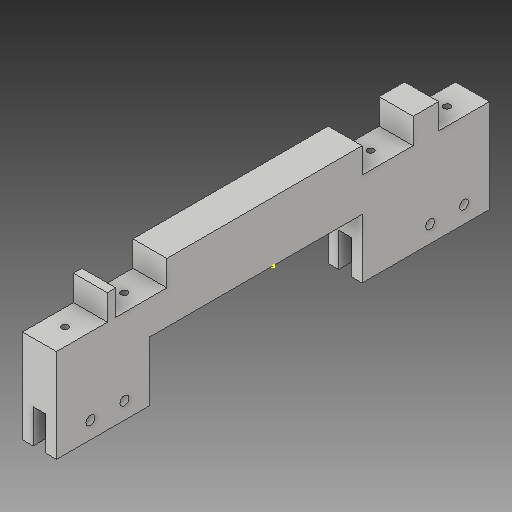
# Autodesk Inventor part: RailSlideLeftSide
Saved by Autodesk Inventor 2017 SP1 (Build 210196100, 196)
## iProperties
Created: 2016-02-14
Part Number: RailSlideLeftSide
Material: Generic
Document SubType Name: Modeling
Designer: steele
Density: 1 g/cm^3
Appearance: Default
Author: steele
Autodesk Inventor part; units mm, degrees
ref_plane "YZ Plane" through (0, 0, 0) normal (1, 0, 0) x (0, 1, 0)
ref_plane "XZ Plane" through (0, 0, 0) normal (0, 1, 0) x (-1, 0, 0)
ref_plane "XY Plane" through (0, 0, 0) normal (0, 0, 1) x (1, 0, 0)
sketch "Sketch1" plane through (0, 0, 0) normal (1, 0, 0) x (0, 1, 0)
  line L0 (-44.45, 161.925) -> (-44.45, -161.925)
  line L1 (-44.45, -161.925) -> (44.45, -161.925)
  line L2 (44.45, -161.925) -> (44.45, 161.925)
  line L3 (44.45, 161.925) -> (-44.45, 161.925)
  line L4 (-44.45, 161.925) -> (44.45, -161.925) construction
  line L5 (-44.45, -161.925) -> (44.45, 161.925) construction
  point P0 (0, 0)
  dimension "d0" = 323.85
  dimension "d1" = 88.9
  constraints: 12 end point, 2 midpoint, 2 parallel, 1 perpendicular, 1 vertical
  measures "d0" distance of L1.end L2.end
  measures "d1" distance of L2.end L0.start
extrude "Extrusion1" add sketch "Sketch1" along normal mid plane 25.4
sketch "Sketch2" plane through (12.7, 0, 0) normal (1, 0, 0) x (0, 0, -1)
  line L0 (-161.925, -44.45) -> (161.925, -44.45) projected
  line L1 (-92.075, -44.45) -> (66.675, -44.45)
  line L2 (66.675, -44.45) -> (66.675, 0)
  line L3 (66.675, 0) -> (-92.075, 0)
  line L4 (-92.075, 0) -> (-92.075, -44.45)
  line L5 (-161.925, 44.45) -> (-161.925, -44.45) projected
  point P0 (0, 0)
  dimension "d4" = 158.75
  dimension "d5" = 44.45
  dimension "d6" = 69.85
  constraints: 8 end point, 2 parallel, 1 horizontal, 1 perpendicular, 1 point on line
  measures "d4" distance of L2.end L3.end
  measures "d5" distance between parallel lines of L0 L3
  measures "d6" distance between parallel lines of L4 L5
extrude "Extrusion2" cut sketch "Sketch2" against normal through all
sketch "Sketch4" plane through (-12.7, -44.45, 161.925) normal (0, 0, 1) x (1, 0, 0)
  line L0 (7.9375, 0) -> (17.4625, 0)
  line L1 (17.4625, 0) -> (17.4625, 25.4)
  line L2 (17.4625, 25.4) -> (7.9375, 25.4)
  line L3 (7.9375, 25.4) -> (7.9375, 0)
  line L4 (25.4, 0) -> (0, 0) projected
  point P0 (12.7, 44.45)
  dimension "d11" = 4.7625
  dimension "d12" = 4.7625
  dimension "d13" = 25.4
  constraints: 8 end point, 2 parallel, 1 collinear, 1 horizontal, 1 perpendicular
  measures "d11" distance from line of point (12.7, 44.45) L3
  measures "d12" distance from line of point (12.7, 44.45) L1
  measures "d13" distance of L2.end L0.start
extrude "Extrusion3" cut sketch "Sketch4" against normal through all
sketch "Sketch6" plane through (12.7, 0, 0) normal (1, 0, 0) x (0, 0, -1)
  point P0 (0, 0)
sketch "Sketch7" plane through (12.7, 0, 0) normal (1, 0, 0) x (0, 0, -1)
  line L0 (-161.925, 44.45) -> (-161.925, -44.45) projected
  line L1 (-161.925, -44.45) -> (-161.925, 44.45) construction
  line L2 (-161.925, -31.75) -> (161.925, -31.75) construction
  line L3 (161.925, 44.45) -> (161.925, -44.45) construction
  point P0 (0, 0)
  point P1 (-136.525, -31.75)
  point P2 (-111.125, -31.75)
  point P3 (117.475, -31.75)
  point P4 (142.875, -31.75)
  dimension "d16" = 12.7
  dimension "d17" = 25.4
  dimension "d18" = 25.4
  dimension "d19" = 279.4
  dimension "d20" = 25.4
  constraints: 6 point on line, 2 end point, 1 horizontal
  measures "d16" distance from line of L2 L0.end
  measures "d17" distance of point (-111.125, -31.75) point (-136.525, -31.75)
  measures "d18" distance from line of L0 point (-136.525, -31.75)
  measures "d19" distance from line of point (117.475, -31.75) L0
  measures "d20" distance of point (142.875, -31.75) point (117.475, -31.75)
hole "Hole1" at (12.7, -31.75, 136.525) at (12.7, -31.75, 111.125) at (12.7, -31.75, -117.475) at (12.7, -31.75, -142.875) direction (-1, 0, 0) diameter 6.7564 end through all clearance for "Flat Head Machine Screw (82)" size "1/4" standard "Ansi Unified Screw Threads"
sketch "Sketch8" plane through (12.7, 0, 0) normal (1, 0, 0) x (0, 0, -1)
  line L0 (-161.925, 44.45) -> (-161.925, -44.45) projected
  line L1 (-161.925, 25.4) -> (-123.825, 25.4)
  line L2 (-123.825, 25.4) -> (-123.825, 44.45)
  line L3 (-123.825, 44.45) -> (-161.925, 44.45)
  line L4 (-161.925, 44.45) -> (-161.925, 25.4)
  line L5 (161.925, 44.45) -> (-161.925, 44.45) projected
  line L6 (161.925, 44.45) -> (161.925, -44.45) projected
  line L7 (161.925, 25.4) -> (123.825, 25.4)
  line L8 (123.825, 25.4) -> (123.825, 44.45)
  line L9 (123.825, 44.45) -> (161.925, 44.45)
  line L10 (161.925, 44.45) -> (161.925, 25.4)
  line L11 (-117.475, 44.45) -> (-79.375, 44.45)
  line L12 (-79.375, 44.45) -> (-79.375, 25.4)
  line L13 (-79.375, 25.4) -> (-117.475, 25.4)
  line L14 (-117.475, 25.4) -> (-117.475, 44.45)
  line L15 (104.775, 25.4) -> (66.675, 25.4)
  line L16 (66.675, 25.4) -> (66.675, 44.45)
  line L17 (66.675, 44.45) -> (104.775, 44.45)
  line L18 (104.775, 44.45) -> (104.775, 25.4)
  point P0 (0, 0)
  dimension "d28" = 38.1
  dimension "d29" = 19.05
  dimension "d30" = 6.35
  dimension "d31" = 146.05
  constraints: 32 end point, 8 parallel, 7 collinear, 5 point on line, 4 horizontal, 4 perpendicular
  measures "d28" distance of L1.start L1.end
  measures "d29" distance of L1.end L2.end
  measures "d30" distance between parallel lines of L14 L2
  measures "d31" distance between parallel lines of L16 L12
extrude "Extrusion4" cut sketch "Sketch8" against normal through all
sketch "Sketch9" plane through (12.7, 25.4, 161.925) normal (0, 1, 0) x (1, 0, 0)
  line L0 (-17.4625, 0) -> (-7.9375, 0) construction
  line L1 (-12.7, 0) -> (-12.7, 323.226) construction
  line L2 (0, 0) -> (-25.4, 0) construction
  line L3 (0, 44.45) -> (-25.4, 44.45) construction
  line L4 (0, 228.6) -> (-25.4, 228.6) construction
  line L5 (0, 285.75) -> (-25.4, 285.75) construction
  point P0 (-12.7, 161.925)
  point P1 (-12.7, 19.05)
  point P2 (-12.7, 63.5)
  point P3 (-12.7, 247.65)
  point P4 (-12.7, 304.8)
  dimension "d34" = 19.05
  dimension "d35" = 19.05
  dimension "d36" = 19.05
  dimension "d37" = 19.05
  constraints: 4 point on line, 2 end point, 1 midpoint, 1 vertical
  measures "d34" distance from line of point (-12.7, 19.05) L2
  measures "d35" distance from line of point (-12.7, 63.5) L3
  measures "d36" distance from line of point (-12.7, 247.65) L4
  measures "d37" distance from line of point (-12.7, 304.8) L5
hole "Hole2" at (0, 25.4, 142.875) at (0, 25.4, 98.425) at (0, 25.4, -85.725) at (0, 25.4, -142.875) direction (0, -1, 0) diameter 4.9784 depth 31.75 tip angle 118 thread size "1/4-20 UNC" class "2B" standard "ANSI Unified Screw Threads"
equation "\"d0\" = RailSlideTotalLength"
equation "\"d1\" = RailSlideTotalHeight"
equation "\"d2\" = RailSlideTotalWidth"
equation "\"d4\" = WidthOfCutoutForTransmission"
equation "\"d5\" = heigthOfCutoutForTransmission"
equation "\"d6\" = distanceFromRearToStartOfTransmissionCutout"
equation "\"d7\" = RailSlideTotalWidth"
equation "\"d11\" = 0.5 * cutoutWidth"
equation "\"d12\" = 0.5 * cutoutWidth"
equation "\"d13\" = cutoutHeight"
equation "\"d14\" = RailSlideTotalWidth"
equation "\"d32\" = RailSlideTotalWidth"
equation "\"RailSlideTotalLength\" = 323.85"
equation "\"RailSlideTotalWidth\" = 25.4"
equation "\"RailSlideTotalHeight\" = 88.9"
equation "\"WidthOfCutoutForTransmission\" = 158.75"
equation "\"heigthOfCutoutForTransmission\" = 44.45"
equation "\"distanceFromRearToStartOfTransmissionCutout\" = 69.85"
equation "\"cutoutWidth\" = 9.525"
equation "\"cutoutHeight\" = 25.4"
body "Solid1"
